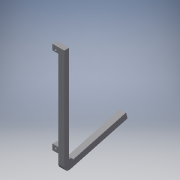
# Autodesk Inventor part: LCD-holder-right
Saved by Autodesk Inventor 2018 (Build 220112000, 112)
## iProperties
Created: 2017-11-15
Part Number: LCD-holder-right
Material: Generic
Document SubType Name: Modeling
Designer: WutchZone
Density: 1 g/cm^3
Appearance: Default
Author: WutchZone
Autodesk Inventor part; units mm, degrees
ref_plane "YZ Plane" through (0, 0, 0) normal (1, 0, 0) x (0, 1, 0)
ref_plane "XZ Plane" through (0, 0, 0) normal (0, 1, 0) x (-1, 0, 0)
ref_plane "XY Plane" through (0, 0, 0) normal (0, 0, 1) x (1, 0, 0)
sketch "Sketch1" plane through (0, 0, 0) normal (0, 0, 1) x (1, 0, 0)
  line L0 (74.45, 62.135) -> (82.45, 62.135)
  line L1 (82.45, 62.135) -> (82.45, -62.135)
  line L2 (82.45, -62.135) -> (74.45, -62.135)
  circle A0 centre (78.45, 57.48) radius 1.55
  circle A1 centre (78.45, -57.48) radius 1.55
  line L3 (78.45, 57.48) -> (78.45, -57.48) construction
  line L4 (74.45, 0) -> (82.45, 0) construction
  line L5 (74.45, 57.48) -> (82.45, 57.48) construction
  line L6 (74.45, 54.48) -> (82.45, 54.48)
  line L7 (74.45, -54.48) -> (82.45, -54.48)
  line L8 (82.45, 62.135) -> (90.45, 62.135)
  line L9 (90.45, 62.135) -> (90.45, -62.135)
  line L10 (90.45, -62.135) -> (82.45, -62.135)
  line L11 (82.45, -62.135) -> (82.45, 62.135)
  line L12 (74.45, -62.135) -> (74.45, -54.48)
  line L13 (74.45, 54.48) -> (74.45, 62.135)
  line L14 (74.45, 54.48) -> (74.45, -54.48) construction
  line L15 (0, 79.555) -> (0, -87.364) construction
  line L16 (74.45, -54.48) -> (82.45, -54.48)
  line L17 (82.45, -54.48) -> (82.45, -62.135)
  line L18 (82.45, -62.135) -> (74.45, -62.135)
  line L19 (74.45, -62.135) -> (74.45, -54.48)
  point P0 (0, 0)
  point P1 (78.45, 0)
  point P2 (78.45, 0)
  point P3 (78.45, 62.135)
  point P4 (86.45, -62.135)
  point P5 (78.45, -62.135)
  dimension "d0" = 124.27
  dimension "d1" = 8
  dimension "d2" = 3.1
  dimension "d3" = 3.1
  dimension "d4" = 114.96
  dimension "d5" = 3
  dimension "d6" = 78.45
  dimension "d7" = 8
  constraints: 40 end point, 9 midpoint, 8 parallel, 5 perpendicular, 4 point on line, 3 horizontal, 2 centre point, 2 horizontal alignment, 2 symmetric about line, 1 collinear, 1 vertical, 1 vertical alignment
  measures "d0" distance of L0.end L1.end
  measures "d1" distance of L0.start L0.end
  measures "d2" diameter of A0
  measures "d3" diameter of A1
  measures "d4" distance of L3.end L3.start
  measures "d5" distance from line of L6 L3.start
  measures "d6" horizontal distance of L3.start point (0, 0)
  measures "d7" distance between parallel lines of L9 L1
extrude "Extrusion3" add sketch "Sketch1" along normal blind 6.5
sketch "Sketch4" plane through (90.45, -62.135, 0) normal (1, 0, 0) x (0, 0, -1)
  line L0 (-6.5, 0) -> (-6.5, 124.27) projected
  line L1 (-6.5, 0) -> (0, 0)
  line L2 (0, 0) -> (0, -12)
  line L3 (0, -12) -> (-6.5, -12)
  line L4 (-6.5, -12) -> (-6.5, 0)
  circle A0 centre (0, -12) radius 6.5
  line L5 (1.6823, -18.2785) -> (78.9564, 2.427)
  line L6 (78.9564, 2.427) -> (76.8858, 10.1544)
  line L7 (76.8858, 10.1544) -> (5.7208, -8.9142)
  point P0 (0, 62.135)
  dimension "d19" = 12
  dimension "d20" = 75
  dimension "d21" = 8
  dimension "d22" = 80
  constraints: 14 end point, 3 parallel, 3 point on circle, 2 coincident, 2 perpendicular, 1 centre point, 1 horizontal, 1 tangent
  measures "d19" distance between parallel lines of L1 L3
  measures "d20" angle of L2 L7
  measures "d21" distance between parallel lines of L7 L5
  measures "d22" distance of L5.end L5.start
extrude "Extrusion4" add sketch "Sketch4" against normal up to surface (8 mm away)
body "Solid2"
